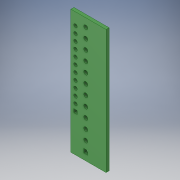
# Autodesk Inventor part: 3_5MM_TO_5_08MM_ADAPTOR_PCB
Saved by Autodesk Inventor 2018 (Build 220112000, 112)
## iProperties
Created: 2018-09-24
Part Number: 3_5MM_TO_5_08MM_ADAPTOR_PCB
Material: ABS Plastic
Document SubType Name: Modeling
Designer: Rich
Density: 1.06 g/cm^3
Appearance: Smooth - Dark Forest Green
Author: Rich
Autodesk Inventor part; units mm, degrees
(part 1 of 13)
ref_plane "YZ Plane" through (0, 0, 0) normal (1, 0, 0) x (0, 1, 0)
ref_plane "XZ Plane" through (0, 0, 0) normal (0, 1, 0) x (-1, 0, 0)
ref_plane "XY Plane" through (0, 0, 0) normal (0, 0, 1) x (1, 0, 0)
sketch "Sketch13" plane through (0, 0, 0) normal (0, 0, 1) x (1, 0, 0)
  line L0 (7.6746, 55.5524) -> (7.2, 55.5524)
  arc A0 (7.2, 55.5524) -> (7.2, 55.5016) centre (7.2, 55.527) ccw
  line L1 (7.7, 55.3688) -> (7.7, 55.6852)
  arc A1 (7.7, 55.6852) -> (7.6492, 55.6852) centre (7.6746, 55.6852) ccw
  line L2 (7.6492, 55.6852) -> (7.6492, 55.3688)
  arc A2 (7.6492, 55.3688) -> (7.7, 55.3688) centre (7.6746, 55.3688) ccw
  line L3 (7.3762, 59.9834) -> (7.218, 60.1416)
  arc A3 (7.218, 60.1416) -> (7.182, 60.1056) centre (7.2, 60.1236) ccw
  line L4 (7.182, 60.1056) -> (7.3402, 59.9474)
  arc A4 (7.3402, 59.9474) -> (7.3762, 59.9834) centre (7.3582, 59.9654) ccw
  line L5 (7.2, 60.0982) -> (7.6746, 60.0982)
  arc A5 (7.6746, 60.0982) -> (7.6746, 60.149) centre (7.6746, 60.1236) ccw
  line L6 (7.6746, 60.149) -> (7.2, 60.149)
  arc A6 (7.2, 60.149) -> (7.2, 60.0982) centre (7.2, 60.1236) ccw
  line L7 (7.7, 59.9654) -> (7.7, 60.2818)
  arc A7 (7.7, 60.2818) -> (7.6492, 60.2818) centre (7.6746, 60.2818) ccw
  line L8 (7.6492, 60.2818) -> (7.6492, 59.9654)
  arc A8 (7.6492, 59.9654) -> (7.7, 59.9654) centre (7.6746, 59.9654) ccw
  line L9 (7.6492, 60.7652) -> (7.6492, 60.4488)
  arc A9 (7.6492, 60.4488) -> (7.7, 60.4488) centre (7.6746, 60.4488) ccw
  line L10 (7.7, 60.4488) -> (7.7, 60.7652)
  arc A10 (7.7, 60.7652) -> (7.6492, 60.7652) centre (7.6746, 60.7661) ccw
  line L11 (7.6926, 60.4668) -> (7.3762, 60.7832)
  arc A11 (7.3762, 60.7832) -> (7.3402, 60.7472) centre (7.3582, 60.7652) ccw
  line L12 (7.3402, 60.7472) -> (7.6566, 60.4308)
  arc A12 (7.6566, 60.4308) -> (7.6926, 60.4668) centre (7.6746, 60.4488) ccw
  line L13 (7.3582, 60.7906) -> (7.2791, 60.7906)
  arc A13 (7.2791, 60.7906) -> (7.2791, 60.7398) centre (7.2791, 60.7652) ccw
  line L14 (7.2791, 60.7398) -> (7.3582, 60.7398)
  arc A14 (7.3582, 60.7398) -> (7.3582, 60.7906) centre (7.3582, 60.7652) ccw
  line L15 (7.2611, 60.7832) -> (7.182, 60.7041)
  arc A15 (7.182, 60.7041) -> (7.218, 60.6681) centre (7.2, 60.6861) ccw
  line L16 (7.218, 60.6681) -> (7.2971, 60.7472)
  arc A16 (7.2971, 60.7472) -> (7.2611, 60.7832) centre (7.2791, 60.7652) ccw
  line L17 (7.1746, 60.6861) -> (7.1746, 60.5279)
  arc A17 (7.1746, 60.5279) -> (7.2254, 60.5279) centre (7.2, 60.5279) ccw
  line L18 (7.2254, 60.5279) -> (7.2254, 60.6861)
  arc A18 (7.2254, 60.6861) -> (7.1746, 60.6861) centre (7.2, 60.6861) ccw
  line L19 (7.182, 60.5099) -> (7.2611, 60.4308)
  arc A19 (7.2611, 60.4308) -> (7.2971, 60.4668) centre (7.2791, 60.4488) ccw
  line L20 (7.2971, 60.4668) -> (7.218, 60.5459)
  arc A20 (7.218, 60.5459) -> (7.182, 60.5099) centre (7.2, 60.5279) ccw
  line L21 (7.3762, 4.1034) -> (7.218, 4.2616)
  arc A21 (7.218, 4.2616) -> (7.182, 4.2256) centre (7.2, 4.2436) ccw
  line L22 (7.182, 4.2256) -> (7.3402, 4.0674)
  arc A22 (7.3402, 4.0674) -> (7.3762, 4.1034) centre (7.3582, 4.0854) ccw
  line L23 (7.2, 4.2182) -> (7.6746, 4.2182)
  arc A23 (7.6746, 4.2182) -> (7.6746, 4.269) centre (7.6746, 4.2436) ccw
  line L24 (7.6746, 4.269) -> (7.2, 4.269)
  arc A24 (7.2, 4.269) -> (7.2, 4.2182) centre (7.2, 4.2436) ccw
  line L25 (7.7, 4.0854) -> (7.7, 4.4018)
  arc A25 (7.7, 4.4018) -> (7.6492, 4.4018) centre (7.6746, 4.4018) ccw
  line L26 (7.6492, 4.4018) -> (7.6492, 4.0854)
  arc A26 (7.6492, 4.0854) -> (7.7, 4.0854) centre (7.6746, 4.0854) ccw
  line L27 (7.6492, 9.4818) -> (7.6492, 9.1654)
  arc A27 (7.6492, 9.1654) -> (7.7, 9.1654) centre (7.6746, 9.1654) ccw
  line L28 (7.7, 9.1654) -> (7.7, 9.4818)
  arc A28 (7.7, 9.4818) -> (7.6492, 9.4818) centre (7.6746, 9.4827) ccw
  line L29 (7.6926, 9.1834) -> (7.3762, 9.4998)
  arc A29 (7.3762, 9.4998) -> (7.3402, 9.4638) centre (7.3582, 9.4818) ccw
  line L30 (7.3402, 9.4638) -> (7.6566, 9.1474)
  arc A30 (7.6566, 9.1474) -> (7.6926, 9.1834) centre (7.6746, 9.1654) ccw
  line L31 (7.3582, 9.5072) -> (7.2791, 9.5072)
  arc A31 (7.2791, 9.5072) -> (7.2791, 9.4564) centre (7.2791, 9.4818) ccw
  line L32 (7.2791, 9.4564) -> (7.3582, 9.4564)
  arc A32 (7.3582, 9.4564) -> (7.3582, 9.5072) centre (7.3582, 9.4818) ccw
  line L33 (7.2611, 9.4998) -> (7.182, 9.4207)
  arc A33 (7.182, 9.4207) -> (7.218, 9.3847) centre (7.2, 9.4027) ccw
  line L34 (7.218, 9.3847) -> (7.2971, 9.4638)
  arc A34 (7.2971, 9.4638) -> (7.2611, 9.4998) centre (7.2791, 9.4818) ccw
  line L35 (7.1746, 9.4027) -> (7.1746, 9.2445)
  arc A35 (7.1746, 9.2445) -> (7.2254, 9.2445) centre (7.2, 9.2445) ccw
  line L36 (7.2254, 9.2445) -> (7.2254, 9.4027)
  arc A36 (7.2254, 9.4027) -> (7.1746, 9.4027) centre (7.2, 9.4027) ccw
  line L37 (7.182, 9.2265) -> (7.2611, 9.1474)
  arc A37 (7.2611, 9.1474) -> (7.2971, 9.1834) centre (7.2791, 9.1654) ccw
  line L38 (7.2971, 9.1834) -> (7.218, 9.2625)
  arc A38 (7.218, 9.2625) -> (7.182, 9.2265) centre (7.2, 9.2445) ccw
  line L39 (7.2971, 14.2634) -> (7.218, 14.3425)
  arc A39 (7.218, 14.3425) -> (7.182, 14.3065) centre (7.2, 14.3245) ccw
  line L40 (7.182, 14.3065) -> (7.2611, 14.2274)
  arc A40 (7.2611, 14.2274) -> (7.2971, 14.2634) centre (7.2791, 14.2454) ccw
  line L41 (7.2254, 14.3245) -> (7.2254, 14.4827)
  arc A41 (7.2254, 14.4827) -> (7.1746, 14.4827) centre (7.2, 14.4827) ccw
  line L42 (7.1746, 14.4827) -> (7.1746, 14.3245)
  arc A42 (7.1746, 14.3245) -> (7.2254, 14.3245) centre (7.2, 14.3245) ccw
  line L43 (7.218, 14.4647) -> (7.2971, 14.5438)
  arc A43 (7.2971, 14.5438) -> (7.2611, 14.5798) centre (7.2791, 14.5618) ccw
  line L44 (7.2611, 14.5798) -> (7.182, 14.5007)
  arc A44 (7.182, 14.5007) -> (7.218, 14.4647) centre (7.2, 14.4827) ccw
  line L45 (7.2791, 14.5364) -> (7.3582, 14.5364)
  arc A45 (7.3582, 14.5364) -> (7.3582, 14.5872) centre (7.3582, 14.5618) ccw
  line L46 (7.3582, 14.5872) -> (7.2791, 14.5872)
  arc A46 (7.2791, 14.5872) -> (7.2791, 14.5364) centre (7.2791, 14.5618) ccw
  line L47 (7.3402, 14.5438) -> (7.4193, 14.4647)
  arc A47 (7.4193, 14.4647) -> (7.4553, 14.5007) centre (7.4373, 14.4827) ccw
  line L48 (7.4553, 14.5007) -> (7.3762, 14.5798)
  arc A48 (7.3762, 14.5798) -> (7.3402, 14.5438) centre (7.3582, 14.5618) ccw
  line L49 (7.4119, 14.4827) -> (7.4119, 14.4036)
  arc A49 (7.4119, 14.4036) -> (7.4627, 14.4036) centre (7.4373, 14.4036) ccw
  line L50 (7.4627, 14.4036) -> (7.4627, 14.4827)
  arc A50 (7.4627, 14.4827) -> (7.4119, 14.4827) centre (7.4373, 14.4827) ccw
  line L51 (7.4553, 14.4647) -> (7.5344, 14.5438)
  arc A51 (7.5344, 14.5438) -> (7.4984, 14.5798) centre (7.5164, 14.5618) ccw
  line L52 (7.4984, 14.5798) -> (7.4193, 14.5007)
  arc A52 (7.4193, 14.5007) -> (7.4553, 14.4647) centre (7.4373, 14.4827) ccw
  line L53 (7.5164, 14.5364) -> (7.5955, 14.5364)
  arc A53 (7.5955, 14.5364) -> (7.5955, 14.5872) centre (7.5955, 14.5618) ccw
  line L54 (7.5955, 14.5872) -> (7.5164, 14.5872)
  arc A54 (7.5164, 14.5872) -> (7.5164, 14.5364) centre (7.5164, 14.5618) ccw
  line L55 (7.5775, 14.5438) -> (7.6566, 14.4647)
  arc A55 (7.6566, 14.4647) -> (7.6926, 14.5007) centre (7.6746, 14.4827) ccw
  line L56 (7.6926, 14.5007) -> (7.6135, 14.5798)
  arc A56 (7.6135, 14.5798) -> (7.5775, 14.5438) centre (7.5955, 14.5618) ccw
  line L57 (7.6492, 14.4827) -> (7.6492, 14.3245)
  arc A57 (7.6492, 14.3245) -> (7.7, 14.3245) centre (7.6746, 14.3245) ccw
  line L58 (7.7, 14.3245) -> (7.7, 14.4827)
  arc A58 (7.7, 14.4827) -> (7.6492, 14.4827) centre (7.6746, 14.4827) ccw
  line L59 (7.6566, 14.3425) -> (7.5775, 14.2634)
  arc A59 (7.5775, 14.2634) -> (7.6135, 14.2274) centre (7.5955, 14.2454) ccw
  line L60 (7.6135, 14.2274) -> (7.6926, 14.3065)
  arc A60 (7.6926, 14.3065) -> (7.6566, 14.3425) centre (7.6746, 14.3245) ccw
  line L61 (7.6746, 19.5881) -> (7.2, 19.5881)
  arc A61 (7.2, 19.5881) -> (7.2, 19.5373) centre (7.2, 19.5627) ccw
  line L62 (7.2, 19.5373) -> (7.6746, 19.5373)
  arc A62 (7.6746, 19.5373) -> (7.6746, 19.5881) centre (7.6746, 19.5627) ccw
  line L63 (7.182, 19.5447) -> (7.4193, 19.3074)
  arc A63 (7.4193, 19.3074) -> (7.4553, 19.3434) centre (7.4373, 19.3254) ccw
  line L64 (7.4553, 19.3434) -> (7.218, 19.5807)
  arc A64 (7.218, 19.5807) -> (7.182, 19.5447) centre (7.2, 19.5627) ccw
  line L65 (7.4627, 19.3254) -> (7.4627, 19.6418)
  arc A65 (7.4627, 19.6418) -> (7.4119, 19.6418) centre (7.4373, 19.6418) ccw
  line L66 (7.4119, 19.6418) -> (7.4119, 19.3254)
  arc A66 (7.4119, 19.3254) -> (7.4627, 19.3254) centre (7.4373, 19.3254) ccw
  line L67 (7.1746, 24.7218) -> (7.1746, 24.4054)
  arc A67 (7.1746, 24.4054) -> (7.2254, 24.4054) centre (7.2, 24.4054) ccw
  line L68 (7.2254, 24.4054) -> (7.2254, 24.7218)
  arc A68 (7.2254, 24.7218) -> (7.1746, 24.7218) centre (7.2, 24.7218) ccw
  line L69 (7.2, 24.38) -> (7.4373, 24.38)
  arc A69 (7.4373, 24.38) -> (7.4373, 24.4308) centre (7.4373, 24.4054) ccw
  line L70 (7.4373, 24.4308) -> (7.2, 24.4308)
  arc A70 (7.2, 24.4308) -> (7.2, 24.38) centre (7.2, 24.4054) ccw
  line L71 (7.46, 24.4168) -> (7.3809, 24.575)
  arc A71 (7.3809, 24.575) -> (7.3355, 24.5522) centre (7.3582, 24.5636) ccw
  line L72 (7.3355, 24.5522) -> (7.4146, 24.394)
  arc A72 (7.4146, 24.394) -> (7.46, 24.4168) centre (7.4373, 24.4054) ccw
  line L73 (7.3836, 24.5636) -> (7.3836, 24.6427)
  arc A73 (7.3836, 24.6427) -> (7.3328, 24.6427) centre (7.3582, 24.6427) ccw
  line L74 (7.3328, 24.6427) -> (7.3328, 24.5636)
  arc A74 (7.3328, 24.5636) -> (7.3836, 24.5636) centre (7.3582, 24.5636) ccw
  line L75 (7.3762, 24.6247) -> (7.4553, 24.7038)
  arc A75 (7.4553, 24.7038) -> (7.4193, 24.7398) centre (7.4373, 24.7218) ccw
  line L76 (7.4193, 24.7398) -> (7.3402, 24.6607)
  arc A76 (7.3402, 24.6607) -> (7.3762, 24.6247) centre (7.3582, 24.6427) ccw
  line L77 (7.4373, 24.6964) -> (7.5955, 24.6964)
  arc A77 (7.5955, 24.6964) -> (7.5955, 24.7472) centre (7.5955, 24.7218) ccw
  line L78 (7.5955, 24.7472) -> (7.4373, 24.7472)
  arc A78 (7.4373, 24.7472) -> (7.4373, 24.6964) centre (7.4373, 24.7218) ccw
  line L79 (7.5775, 24.7038) -> (7.6566, 24.6247)
  arc A79 (7.6566, 24.6247) -> (7.6926, 24.6607) centre (7.6746, 24.6427) ccw
  line L80 (7.6926, 24.6607) -> (7.6135, 24.7398)
  arc A80 (7.6135, 24.7398) -> (7.5775, 24.7038) centre (7.5955, 24.7218) ccw
  line L81 (7.6492, 24.6427) -> (7.6492, 24.4845)
  arc A81 (7.6492, 24.4845) -> (7.7, 24.4845) centre (7.6746, 24.4845) ccw
  line L82 (7.7, 24.4845) -> (7.7, 24.6427)
  arc A82 (7.7, 24.6427) -> (7.6492, 24.6427) centre (7.6746, 24.6427) ccw
  line L83 (7.6566, 24.5025) -> (7.5775, 24.4234)
  arc A83 (7.5775, 24.4234) -> (7.6135, 24.3874) centre (7.5955, 24.4054) ccw
  line L84 (7.6135, 24.3874) -> (7.6926, 24.4665)
  arc A84 (7.6926, 24.4665) -> (7.6566, 24.5025) centre (7.6746, 24.4845) ccw
  line L85 (7.1773, 29.7904) -> (7.2564, 29.6322)
  arc A85 (7.2564, 29.6322) -> (7.3018, 29.655) centre (7.2791, 29.6436) ccw
  line L86 (7.3018, 29.655) -> (7.2227, 29.8132)
  arc A86 (7.2227, 29.8132) -> (7.1773, 29.7904) centre (7.2, 29.8018) ccw
  line L87 (7.2611, 29.6256) -> (7.4193, 29.4674)
  arc A87 (7.4193, 29.4674) -> (7.4553, 29.5034) centre (7.4373, 29.4854) ccw
  line L88 (7.4553, 29.5034) -> (7.2971, 29.6616)
  arc A88 (7.2971, 29.6616) -> (7.2611, 29.6256) centre (7.2791, 29.6436) ccw
  line L89 (7.4373, 29.46) -> (7.5955, 29.46)
  arc A89 (7.5955, 29.46) -> (7.5955, 29.5108) centre (7.5955, 29.4854) ccw
  line L90 (7.5955, 29.5108) -> (7.4373, 29.5108)
  arc A90 (7.4373, 29.5108) -> (7.4373, 29.46) centre (7.4373, 29.4854) ccw
  line L91 (7.6135, 29.4674) -> (7.6926, 29.5465)
  arc A91 (7.6926, 29.5465) -> (7.6566, 29.5825) centre (7.6746, 29.5645) ccw
  line L92 (7.6566, 29.5825) -> (7.5775, 29.5034)
  arc A92 (7.5775, 29.5034) -> (7.6135, 29.4674) centre (7.5955, 29.4854) ccw
  line L93 (7.7, 29.5645) -> (7.7, 29.7227)
  arc A93 (7.7, 29.7227) -> (7.6492, 29.7227) centre (7.6746, 29.7227) ccw
  line L94 (7.6492, 29.7227) -> (7.6492, 29.5645)
  arc A94 (7.6492, 29.5645) -> (7.7, 29.5645) centre (7.6746, 29.5645) ccw
  line L95 (7.6926, 29.7407) -> (7.6135, 29.8198)
  arc A95 (7.6135, 29.8198) -> (7.5775, 29.7838) centre (7.5955, 29.8018) ccw
  line L96 (7.5775, 29.7838) -> (7.6566, 29.7047)
  arc A96 (7.6566, 29.7047) -> (7.6926, 29.7407) centre (7.6746, 29.7227) ccw
  line L97 (7.5955, 29.8272) -> (7.5164, 29.8272)
  arc A97 (7.5164, 29.8272) -> (7.5164, 29.7764) centre (7.5164, 29.8018) ccw
  line L98 (7.5164, 29.7764) -> (7.5955, 29.7764)
  arc A98 (7.5955, 29.7764) -> (7.5955, 29.8272) centre (7.5955, 29.8018) ccw
  line L99 (7.4984, 29.8198) -> (7.4193, 29.7407)
  arc A99 (7.4193, 29.7407) -> (7.4553, 29.7047) centre (7.4373, 29.7227) ccw
  line L100 (7.4553, 29.7047) -> (7.5344, 29.7838)
  arc A100 (7.5344, 29.7838) -> (7.4984, 29.8198) centre (7.5164, 29.8018) ccw
  line L101 (7.4119, 29.7227) -> (7.4119, 29.4854)
  arc A101 (7.4119, 29.4854) -> (7.4627, 29.4854) centre (7.4373, 29.4854) ccw
  line L102 (7.4627, 29.4854) -> (7.4627, 29.7227)
  arc A102 (7.4627, 29.7227) -> (7.4119, 29.7227) centre (7.4373, 29.7227) ccw
  line L103 (7.2254, 34.5654) -> (7.2254, 34.8818)
  arc A103 (7.2254, 34.8818) -> (7.1746, 34.8818) centre (7.2, 34.8818) ccw
  line L104 (7.1746, 34.8818) -> (7.1746, 34.5654)
  arc A104 (7.1746, 34.5654) -> (7.2254, 34.5654) centre (7.2, 34.5654) ccw
  line L105 (7.2, 34.8564) -> (7.2791, 34.8564)
  arc A105 (7.2791, 34.8564) -> (7.2791, 34.9072) centre (7.2791, 34.8818) ccw
  line L106 (7.2791, 34.9072) -> (7.2, 34.9072)
  arc A106 (7.2, 34.9072) -> (7.2, 34.8564) centre (7.2, 34.8818) ccw
  line L107 (7.2611, 34.8638) -> (7.5775, 34.5474)
  arc A107 (7.5775, 34.5474) -> (7.6135, 34.5834) centre (7.5955, 34.5654) ccw
  line L108 (7.6135, 34.5834) -> (7.2971, 34.8998)
  arc A108 (7.2971, 34.8998) -> (7.2611, 34.8638) centre (7.2791, 34.8818) ccw
  line L109 (7.5955, 34.54) -> (7.6746, 34.54)
  arc A109 (7.6746, 34.54) -> (7.6746, 34.5908) centre (7.6746, 34.5654) ccw
  line L110 (7.6746, 34.5908) -> (7.5955, 34.5908)
  arc A110 (7.5955, 34.5908) -> (7.5955, 34.54) centre (7.5955, 34.5654) ccw
  line L111 (7.2971, 39.6634) -> (7.218, 39.7425)
  arc A111 (7.218, 39.7425) -> (7.182, 39.7065) centre (7.2, 39.7245) ccw
  line L112 (7.182, 39.7065) -> (7.2611, 39.6274)
  arc A112 (7.2611, 39.6274) -> (7.2971, 39.6634) centre (7.2791, 39.6454) ccw
  line L113 (7.2254, 39.7245) -> (7.2254, 39.8827)
  arc A113 (7.2254, 39.8827) -> (7.1746, 39.8827) centre (7.2, 39.8827) ccw
  line L114 (7.1746, 39.8827) -> (7.1746, 39.7245)
  arc A114 (7.1746, 39.7245) -> (7.2254, 39.7245) centre (7.2, 39.7245) ccw
  line L115 (7.218, 39.8647) -> (7.2971, 39.9438)
  arc A115 (7.2971, 39.9438) -> (7.2611, 39.9798) centre (7.2791, 39.9618) ccw
  line L116 (7.2611, 39.9798) -> (7.182, 39.9007)
  arc A116 (7.182, 39.9007) -> (7.218, 39.8647) centre (7.2, 39.8827) ccw
  line L117 (7.2791, 39.9364) -> (7.3582, 39.9364)
  arc A117 (7.3582, 39.9364) -> (7.3582, 39.9872) centre (7.3582, 39.9618) ccw
  line L118 (7.3582, 39.9872) -> (7.2791, 39.9872)
  arc A118 (7.2791, 39.9872) -> (7.2791, 39.9364) centre (7.2791, 39.9618) ccw
  line L119 (7.3402, 39.9438) -> (7.4193, 39.8647)
  arc A119 (7.4193, 39.8647) -> (7.4553, 39.9007) centre (7.4373, 39.8827) ccw
  line L120 (7.4553, 39.9007) -> (7.3762, 39.9798)
  arc A120 (7.3762, 39.9798) -> (7.3402, 39.9438) centre (7.3582, 39.9618) ccw
  line L121 (7.4553, 39.8647) -> (7.5344, 39.9438)
  arc A121 (7.5344, 39.9438) -> (7.4984, 39.9798) centre (7.5164, 39.9618) ccw
  line L122 (7.4984, 39.9798) -> (7.4193, 39.9007)
  arc A122 (7.4193, 39.9007) -> (7.4553, 39.8647) centre (7.4373, 39.8827) ccw
  line L123 (7.5164, 39.9364) -> (7.5955, 39.9364)
  arc A123 (7.5955, 39.9364) -> (7.5955, 39.9872) centre (7.5955, 39.9618) ccw
  line L124 (7.5955, 39.9872) -> (7.5164, 39.9872)
  arc A124 (7.5164, 39.9872) -> (7.5164, 39.9364) centre (7.5164, 39.9618) ccw
  line L125 (7.5775, 39.9438) -> (7.6566, 39.8647)
  arc A125 (7.6566, 39.8647) -> (7.6926, 39.9007) centre (7.6746, 39.8827) ccw
  line L126 (7.6926, 39.9007) -> (7.6135, 39.9798)
  arc A126 (7.6135, 39.9798) -> (7.5775, 39.9438) centre (7.5955, 39.9618) ccw
  line L127 (7.6492, 39.8827) -> (7.6492, 39.7245)
  arc A127 (7.6492, 39.7245) -> (7.7, 39.7245) centre (7.6746, 39.7245) ccw
  line L128 (7.7, 39.7245) -> (7.7, 39.8827)
  arc A128 (7.7, 39.8827) -> (7.6492, 39.8827) centre (7.6746, 39.8827) ccw
  line L129 (7.6566, 39.7425) -> (7.5775, 39.6634)
  arc A129 (7.5775, 39.6634) -> (7.6135, 39.6274) centre (7.5955, 39.6454) ccw
  line L130 (7.6135, 39.6274) -> (7.6926, 39.7065)
  arc A130 (7.6926, 39.7065) -> (7.6566, 39.7425) centre (7.6746, 39.7245) ccw
  line L131 (7.5955, 39.6708) -> (7.5164, 39.6708)
  arc A131 (7.5164, 39.6708) -> (7.5164, 39.62) centre (7.5164, 39.6454) ccw
  line L132 (7.5164, 39.62) -> (7.5955, 39.62)
  arc A132 (7.5955, 39.62) -> (7.5955, 39.6708) centre (7.5955, 39.6454) ccw
  line L133 (7.5344, 39.6634) -> (7.4553, 39.7425)
  arc A133 (7.4553, 39.7425) -> (7.4193, 39.7065) centre (7.4373, 39.7245) ccw
  line L134 (7.4193, 39.7065) -> (7.4984, 39.6274)
  arc A134 (7.4984, 39.6274) -> (7.5344, 39.6634) centre (7.5164, 39.6454) ccw
  line L135 (7.4193, 39.7425) -> (7.3402, 39.6634)
  arc A135 (7.3402, 39.6634) -> (7.3762, 39.6274) centre (7.3582, 39.6454) ccw
  line L136 (7.3762, 39.6274) -> (7.4553, 39.7065)
  arc A136 (7.4553, 39.7065) -> (7.4193, 39.7425) centre (7.4373, 39.7245) ccw
  line L137 (7.3582, 39.6708) -> (7.2791, 39.6708)
  arc A137 (7.2791, 39.6708) -> (7.2791, 39.62) centre (7.2791, 39.6454) ccw
  line L138 (7.2791, 39.62) -> (7.3582, 39.62)
  arc A138 (7.3582, 39.62) -> (7.3582, 39.6708) centre (7.3582, 39.6454) ccw
  line L139 (7.4627, 39.7245) -> (7.4627, 39.8827)
  arc A139 (7.4627, 39.8827) -> (7.4119, 39.8827) centre (7.4373, 39.8827) ccw
  line L140 (7.4119, 39.8827) -> (7.4119, 39.7245)
  arc A140 (7.4119, 39.7245) -> (7.4627, 39.7245) centre (7.4373, 39.7245) ccw
  line L141 (7.6135, 44.7074) -> (7.6926, 44.7865)
  arc A141 (7.6926, 44.7865) -> (7.6566, 44.8225) centre (7.6746, 44.8045) ccw
  line L142 (7.6566, 44.8225) -> (7.5775, 44.7434)
  arc A142 (7.5775, 44.7434) -> (7.6135, 44.7074) centre (7.5955, 44.7254) ccw
  line L143 (7.7, 44.8045) -> (7.7, 44.9627)
  arc A143 (7.7, 44.9627) -> (7.6492, 44.9627) centre (7.6746, 44.9627) ccw
  line L144 (7.6492, 44.9627) -> (7.6492, 44.8045)
  arc A144 (7.6492, 44.8045) -> (7.7, 44.8045) centre (7.6746, 44.8045) ccw
  line L145 (7.6926, 44.9807) -> (7.6135, 45.0598)
  arc A145 (7.6135, 45.0598) -> (7.5775, 45.0238) centre (7.5955, 45.0418) ccw
  line L146 (7.5775, 45.0238) -> (7.6566, 44.9447)
  arc A146 (7.6566, 44.9447) -> (7.6926, 44.9807) centre (7.6746, 44.9627) ccw
  line L147 (7.5955, 45.0672) -> (7.2791, 45.0672)
  arc A147 (7.2791, 45.0672) -> (7.2791, 45.0164) centre (7.2791, 45.0418) ccw
  line L148 (7.2791, 45.0164) -> (7.5955, 45.0164)
  arc A148 (7.5955, 45.0164) -> (7.5955, 45.0672) centre (7.5955, 45.0418) ccw
  line L149 (7.2611, 45.0598) -> (7.182, 44.9807)
  arc A149 (7.182, 44.9807) -> (7.218, 44.9447) centre (7.2, 44.9627) ccw
  line L150 (7.218, 44.9447) -> (7.2971, 45.0238)
  arc A150 (7.2971, 45.0238) -> (7.2611, 45.0598) centre (7.2791, 45.0418) ccw
  line L151 (7.1746, 44.9627) -> (7.1746, 44.8045)
  arc A151 (7.1746, 44.8045) -> (7.2254, 44.8045) centre (7.2, 44.8045) ccw
  line L152 (7.2254, 44.8045) -> (7.2254, 44.9627)
  arc A152 (7.2254, 44.9627) -> (7.1746, 44.9627) centre (7.2, 44.9627) ccw
  line L153 (7.182, 44.7865) -> (7.2611, 44.7074)
  arc A153 (7.2611, 44.7074) -> (7.2971, 44.7434) centre (7.2791, 44.7254) ccw
  line L154 (7.2971, 44.7434) -> (7.218, 44.8225)
  arc A154 (7.218, 44.8225) -> (7.182, 44.7865) centre (7.2, 44.8045) ccw
  line L155 (7.2791, 44.7) -> (7.3582, 44.7)
  arc A155 (7.3582, 44.7) -> (7.3582, 44.7508) centre (7.3582, 44.7254) ccw
  line L156 (7.3582, 44.7508) -> (7.2791, 44.7508)
  arc A156 (7.2791, 44.7508) -> (7.2791, 44.7) centre (7.2791, 44.7254) ccw
  line L157 (7.3762, 44.7074) -> (7.4553, 44.7865)
  arc A157 (7.4553, 44.7865) -> (7.4193, 44.8225) centre (7.4373, 44.8045) ccw
  line L158 (7.4193, 44.8225) -> (7.3402, 44.7434)
  arc A158 (7.3402, 44.7434) -> (7.3762, 44.7074) centre (7.3582, 44.7254) ccw
  line L159 (7.4627, 44.8045) -> (7.4627, 45.0418)
  arc A159 (7.4627, 45.0418) -> (7.4119, 45.0418) centre (7.4373, 45.0418) ccw
  line L160 (7.4119, 45.0418) -> (7.4119, 44.8045)
  arc A160 (7.4119, 44.8045) -> (7.4627, 44.8045) centre (7.4373, 44.8045) ccw
  line L161 (7.3762, 49.8234) -> (7.218, 49.9816)
  arc A161 (7.218, 49.9816) -> (7.182, 49.9456) centre (7.2, 49.9636) ccw
  line L162 (7.182, 49.9456) -> (7.3402, 49.7874)
  arc A162 (7.3402, 49.7874) -> (7.3762, 49.8234) centre (7.3582, 49.8054) ccw
  line L163 (7.2, 49.9382) -> (7.6746, 49.9382)
  arc A163 (7.6746, 49.9382) -> (7.6746, 49.989) centre (7.6746, 49.9636) ccw
  line L164 (7.6746, 49.989) -> (7.2, 49.989)
  arc A164 (7.2, 49.989) -> (7.2, 49.9382) centre (7.2, 49.9636) ccw
  line L165 (7.7, 49.8054) -> (7.7, 50.1218)
  arc A165 (7.7, 50.1218) -> (7.6492, 50.1218) centre (7.6746, 50.1218) ccw
  line L166 (7.6492, 50.1218) -> (7.6492, 49.8054)
  arc A166 (7.6492, 49.8054) -> (7.7, 49.8054) centre (7.6746, 49.8054) ccw
  line L167 (7.5955, 50.3142) -> (7.2791, 50.3142)
  arc A167 (7.2791, 50.3142) -> (7.2791, 50.2634) centre (7.2791, 50.2888) ccw
  line L168 (7.2791, 50.2634) -> (7.5955, 50.2634)
  arc A168 (7.5955, 50.2634) -> (7.5955, 50.3142) centre (7.5955, 50.2888) ccw
  line L169 (7.2971, 50.3068) -> (7.218, 50.3859)
  arc A169 (7.218, 50.3859) -> (7.182, 50.3499) centre (7.2, 50.3679) ccw
  line L170 (7.182, 50.3499) -> (7.2611, 50.2708)
  arc A170 (7.2611, 50.2708) -> (7.2971, 50.3068) centre (7.2791, 50.2888) ccw
  line L171 (7.2254, 50.3679) -> (7.2254, 50.5261)
  arc A171 (7.2254, 50.5261) -> (7.1746, 50.5261) centre (7.2, 50.5261) ccw
  line L172 (7.1746, 50.5261) -> (7.1746, 50.3679)
  arc A172 (7.1746, 50.3679) -> (7.2254, 50.3679) centre (7.2, 50.3679) ccw
  line L173 (7.218, 50.5081) -> (7.2971, 50.5872)
  arc A173 (7.2971, 50.5872) -> (7.2611, 50.6232) centre (7.2791, 50.6052) ccw
  line L174 (7.2611, 50.6232) -> (7.182, 50.5441)
  arc A174 (7.182, 50.5441) -> (7.218, 50.5081) centre (7.2, 50.5261) ccw
  line L175 (7.2791, 50.5798) -> (7.5955, 50.5798)
  arc A175 (7.5955, 50.5798) -> (7.5955, 50.6306) centre (7.5955, 50.6052) ccw
  line L176 (7.5955, 50.6306) -> (7.2791, 50.6306)
  arc A176 (7.2791, 50.6306) -> (7.2791, 50.5798) centre (7.2791, 50.6052) ccw
  line L177 (7.5775, 50.5872) -> (7.6566, 50.5081)
  arc A177 (7.6566, 50.5081) -> (7.6926, 50.5441) centre (7.6746, 50.5261) ccw
  line L178 (7.6926, 50.5441) -> (7.6135, 50.6232)
  arc A178 (7.6135, 50.6232) -> (7.5775, 50.5872) centre (7.5955, 50.6052) ccw
  line L179 (7.6492, 50.5261) -> (7.6492, 50.3679)
  arc A179 (7.6492, 50.3679) -> (7.7, 50.3679) centre (7.6746, 50.3679) ccw
  line L180 (7.7, 50.3679) -> (7.7, 50.5261)
  arc A180 (7.7, 50.5261) -> (7.6492, 50.5261) centre (7.6746, 50.5261) ccw
  line L181 (7.6566, 50.3859) -> (7.5775, 50.3068)
  arc A181 (7.5775, 50.3068) -> (7.6135, 50.2708) centre (7.5955, 50.2888) ccw
  line L182 (7.6135, 50.2708) -> (7.6926, 50.3499)
  arc A182 (7.6926, 50.3499) -> (7.6566, 50.3859) centre (7.6746, 50.3679) ccw
  line L183 (7.6135, 50.3068) -> (7.2971, 50.6232)
  arc A183 (7.2971, 50.6232) -> (7.2611, 50.5872) centre (7.2791, 50.6052) ccw
  line L184 (7.2611, 50.5872) -> (7.5775, 50.2708)
  arc A184 (7.5775, 50.2708) -> (7.6135, 50.3068) centre (7.5955, 50.2888) ccw
  line L185 (7.3762, 54.9034) -> (7.218, 55.0616)
  arc A185 (7.218, 55.0616) -> (7.182, 55.0256) centre (7.2, 55.0436) ccw
  line L186 (7.182, 55.0256) -> (7.3402, 54.8674)
  arc A186 (7.3402, 54.8674) -> (7.3762, 54.9034) centre (7.3582, 54.8854) ccw
  line L187 (7.2, 55.0182) -> (7.6746, 55.0182)
  arc A187 (7.6746, 55.0182) -> (7.6746, 55.069) centre (7.6746, 55.0436) ccw
  line L188 (7.6746, 55.069) -> (7.2, 55.069)
  arc A188 (7.2, 55.069) -> (7.2, 55.0182) centre (7.2, 55.0436) ccw
  line L189 (7.7, 54.8854) -> (7.7, 55.2018)
  arc A189 (7.7, 55.2018) -> (7.6492, 55.2018) centre (7.6746, 55.2018) ccw
  line L190 (7.6492, 55.2018) -> (7.6492, 54.8854)
  arc A190 (7.6492, 54.8854) -> (7.7, 54.8854) centre (7.6746, 54.8854) ccw
  line L191 (7.3762, 55.3868) -> (7.218, 55.545)
  arc A191 (7.218, 55.545) -> (7.182, 55.509) centre (7.2, 55.527) ccw
  line L192 (7.182, 55.509) -> (7.3402, 55.3508)
  arc A192 (7.3402, 55.3508) -> (7.3762, 55.3868) centre (7.3582, 55.3688) ccw
  line L193 (7.2, 55.5016) -> (7.6746, 55.5016)
  arc A193 (7.6746, 55.5016) -> (7.6746, 55.5524) centre (7.6746, 55.527) ccw
  line L194 (17.121, 38.367) -> (8.095, 38.367)
  arc A194 (8.095, 38.367) -> (8.095, 38.241) centre (8.095, 38.304) ccw
  line L195 (1.0789, 38.367) -> (7.0006, 38.367)
  arc A195 (7.0006, 38.367) -> (7.0006, 38.493) centre (7.0006, 38.43) ccw
  line L196 (7.0006, 38.493) -> (1.0789, 38.493)
  arc A196 (1.0789, 38.493) -> (1.0789, 38.367) centre (1.0789, 38.43) ccw
  line L197 (7.637, 38.367) -> (7.7628, 38.367)
  arc A197 (7.7628, 38.367) -> (7.7628, 38.493) centre (7.7628, 38.43) ccw
  line L198 (7.7628, 38.493) -> (7.637, 38.493)
  arc A198 (7.637, 38.493) -> (7.637, 38.367) centre (7.637, 38.43) ccw
  line L199 (8.3992, 38.367) -> (17.121, 38.367)
  arc A199 (17.121, 38.367) -> (17.121, 38.493) centre (17.121, 38.43) ccw
  line L200 (17.121, 38.493) -> (8.3992, 38.493)
  arc A200 (8.3992, 38.493) -> (8.3992, 38.367) centre (8.3992, 38.43) ccw
  line L201 (1.0789, 38.493) -> (6.8307, 38.493)
  arc A201 (6.8307, 38.493) -> (6.8307, 38.619) centre (6.8307, 38.556) ccw
  line L202 (6.8307, 38.619) -> (1.0789, 38.619)
  arc A202 (1.0789, 38.619) -> (1.0789, 38.493) centre (1.0789, 38.556) ccw
  line L203 (7.637, 38.493) -> (7.7628, 38.493)
  arc A203 (7.7628, 38.493) -> (7.7628, 38.619) centre (7.7628, 38.556) ccw
  line L204 (7.7628, 38.619) -> (7.637, 38.619)
  arc A204 (7.637, 38.619) -> (7.637, 38.493) centre (7.637, 38.556) ccw
  line L205 (8.5692, 38.493) -> (17.121, 38.493)
  arc A205 (17.121, 38.493) -> (17.121, 38.619) centre (17.121, 38.556) ccw
  line L206 (17.121, 38.619) -> (8.5692, 38.619)
  arc A206 (8.5692, 38.619) -> (8.5692, 38.493) centre (8.5692, 38.556) ccw
  line L207 (1.0789, 38.619) -> (6.7047, 38.619)
  arc A207 (6.7047, 38.619) -> (6.7047, 38.745) centre (6.7047, 38.682) ccw
  line L208 (6.7047, 38.745) -> (1.0789, 38.745)
  arc A208 (1.0789, 38.745) -> (1.0789, 38.619) centre (1.0789, 38.682) ccw
  line L209 (7.637, 38.619) -> (7.7628, 38.619)
  arc A209 (7.7628, 38.619) -> (7.7628, 38.745) centre (7.7628, 38.682) ccw
  line L210 (7.7628, 38.745) -> (7.637, 38.745)
  arc A210 (7.637, 38.745) -> (7.637, 38.619) centre (7.637, 38.682) ccw
  line L211 (8.6952, 38.619) -> (17.121, 38.619)
  arc A211 (17.121, 38.619) -> (17.121, 38.745) centre (17.121, 38.682) ccw
  line L212 (17.121, 38.745) -> (8.6952, 38.745)
  arc A212 (8.6952, 38.745) -> (8.6952, 38.619) centre (8.6952, 38.682) ccw
  line L213 (1.0789, 38.745) -> (6.5787, 38.745)
  arc A213 (6.5787, 38.745) -> (6.5787, 38.871) centre (6.5787, 38.808) ccw
  line L214 (6.5787, 38.871) -> (1.0789, 38.871)
  arc A214 (1.0789, 38.871) -> (1.0789, 38.745) centre (1.0789, 38.808) ccw
  line L215 (7.637, 38.745) -> (7.7628, 38.745)
  arc A215 (7.7628, 38.745) -> (7.7628, 38.871) centre (7.7628, 38.808) ccw
  line L216 (7.7628, 38.871) -> (7.637, 38.871)
  arc A216 (7.637, 38.871) -> (7.637, 38.745) centre (7.637, 38.808) ccw
  line L217 (8.8212, 38.745) -> (17.121, 38.745)
  arc A217 (17.121, 38.745) -> (17.121, 38.871) centre (17.121, 38.808) ccw
  line L218 (17.121, 38.871) -> (8.8212, 38.871)
  arc A218 (8.8212, 38.871) -> (8.8212, 38.745) centre (8.8212, 38.808) ccw
  line L219 (1.0789, 38.871) -> (6.5044, 38.871)
  arc A219 (6.5044, 38.871) -> (6.5044, 38.997) centre (6.5044, 38.934) ccw
  line L220 (6.5044, 38.997) -> (1.0789, 38.997)
  arc A220 (1.0789, 38.997) -> (1.0789, 38.871) centre (1.0789, 38.934) ccw
  line L221 (7.637, 38.871) -> (7.7628, 38.871)
  arc A221 (7.7628, 38.871) -> (7.7628, 38.997) centre (7.7628, 38.934) ccw
  line L222 (7.7628, 38.997) -> (7.637, 38.997)
  arc A222 (7.637, 38.997) -> (7.637, 38.871) centre (7.637, 38.934) ccw
  line L223 (8.8954, 38.871) -> (17.121, 38.871)
  arc A223 (17.121, 38.871) -> (17.121, 38.997) centre (17.121, 38.934) ccw
  line L224 (17.121, 38.997) -> (8.8954, 38.997)
  arc A224 (8.8954, 38.997) -> (8.8954, 38.871) centre (8.8954, 38.934) ccw
  line L225 (1.0789, 38.997) -> (6.4522, 38.997)
  arc A225 (6.4522, 38.997) -> (6.4522, 39.123) centre (6.4522, 39.06) ccw
  line L226 (6.4522, 39.123) -> (1.0789, 39.123)
  arc A226 (1.0789, 39.123) -> (1.0789, 38.997) centre (1.0789, 39.06) ccw
  line L227 (7.637, 38.997) -> (7.7628, 38.997)
  arc A227 (7.7628, 38.997) -> (7.7628, 39.123) centre (7.7628, 39.06) ccw
  line L228 (7.7628, 39.123) -> (7.637, 39.123)
  arc A228 (7.637, 39.123) -> (7.637, 38.997) centre (7.637, 39.06) ccw
  line L229 (8.9476, 38.997) -> (17.121, 38.997)
  arc A229 (17.121, 38.997) -> (17.121, 39.123) centre (17.121, 39.06) ccw
  line L230 (17.121, 39.123) -> (8.9476, 39.123)
  arc A230 (8.9476, 39.123) -> (8.9476, 38.997) centre (8.9476, 39.06) ccw
  line L231 (1.0789, 39.123) -> (6.4001, 39.123)
  arc A231 (6.4001, 39.123) -> (6.4001, 39.249) centre (6.4001, 39.186) ccw
  line L232 (6.4001, 39.249) -> (1.0789, 39.249)
  arc A232 (1.0789, 39.249) -> (1.0789, 39.123) centre (1.0789, 39.186) ccw
  line L233 (7.637, 39.123) -> (7.7628, 39.123)
  arc A233 (7.7628, 39.123) -> (7.7628, 39.249) centre (7.7628, 39.186) ccw
  line L234 (7.7628, 39.249) -> (7.637, 39.249)
  arc A234 (7.637, 39.249) -> (7.637, 39.123) centre (7.637, 39.186) ccw
  line L235 (8.9997, 39.123) -> (17.121, 39.123)
  arc A235 (17.121, 39.123) -> (17.121, 39.249) centre (17.121, 39.186) ccw
  line L236 (17.121, 39.249) -> (8.9997, 39.249)
  arc A236 (8.9997, 39.249) -> (8.9997, 39.123) centre (8.9997, 39.186) ccw
  line L237 (1.0789, 39.249) -> (6.3479, 39.249)
  arc A237 (6.3479, 39.249) -> (6.3479, 39.375) centre (6.3479, 39.312) ccw
  line L238 (6.3479, 39.375) -> (1.0789, 39.375)
  arc A238 (1.0789, 39.375) -> (1.0789, 39.249) centre (1.0789, 39.312) ccw
  line L239 (7.637, 39.249) -> (7.7628, 39.249)
  arc A239 (7.7628, 39.249) -> (7.7628, 39.375) centre (7.7628, 39.312) ccw
  line L240 (7.7628, 39.375) -> (7.637, 39.375)
  arc A240 (7.637, 39.375) -> (7.637, 39.249) centre (7.637, 39.312) ccw
  line L241 (9.0519, 39.249) -> (17.121, 39.249)
  arc A241 (17.121, 39.249) -> (17.121, 39.375) centre (17.121, 39.312) ccw
  line L242 (17.121, 39.375) -> (9.0519, 39.375)
  arc A242 (9.0519, 39.375) -> (9.0519, 39.249) centre (9.0519, 39.312) ccw
  line L243 (1.0789, 39.375) -> (1.9284, 39.375)
  arc A243 (1.9284, 39.375) -> (1.9284, 39.501) centre (1.9284, 39.438) ccw
  line L244 (1.9284, 39.501) -> (1.0789, 39.501)
  arc A244 (1.0789, 39.501) -> (1.0789, 39.375) centre (1.0789, 39.438) ccw
  line L245 (2.8714, 39.375) -> (6.333, 39.375)
  arc A245 (6.333, 39.375) -> (6.333, 39.501) centre (6.333, 39.438) ccw
  line L246 (6.333, 39.501) -> (2.8714, 39.501)
  arc A246 (2.8714, 39.501) -> (2.8714, 39.375) centre (2.8714, 39.438) ccw
  line L247 (7.637, 39.375) -> (7.7628, 39.375)
  arc A247 (7.7628, 39.375) -> (7.7628, 39.501) centre (7.7628, 39.438) ccw
  line L248 (7.7628, 39.501) -> (7.637, 39.501)
  arc A248 (7.637, 39.501) -> (7.637, 39.375) centre (7.637, 39.438) ccw
  line L249 (9.0669, 39.375) -> (17.121, 39.375)
  arc A249 (17.121, 39.375) -> (17.121, 39.501) centre (17.121, 39.438) ccw
  line L250 (17.121, 39.501) -> (9.0669, 39.501)
  arc A250 (9.0669, 39.501) -> (9.0669, 39.375) centre (9.0669, 39.438) ccw
  line L251 (1.0789, 39.501) -> (1.7085, 39.501)
  arc A251 (1.7085, 39.501) -> (1.7085, 39.627) centre (1.7085, 39.564) ccw
  line L252 (1.7085, 39.627) -> (1.0789, 39.627)
  arc A252 (1.0789, 39.627) -> (1.0789, 39.501) centre (1.0789, 39.564) ccw
  line L253 (3.0914, 39.501) -> (7.6365, 39.501)
  arc A253 (7.6365, 39.501) -> (7.6365, 39.627) centre (7.6365, 39.564) ccw
  line L254 (7.6365, 39.627) -> (3.0914, 39.627)
  arc A254 (3.0914, 39.627) -> (3.0914, 39.501) centre (3.0914, 39.564) ccw
  line L255 (7.7634, 39.501) -> (17.121, 39.501)
  arc A255 (17.121, 39.501) -> (17.121, 39.627) centre (17.121, 39.564) ccw
  line L256 (17.121, 39.627) -> (7.7634, 39.627)
  arc A256 (7.7634, 39.627) -> (7.7634, 39.501) centre (7.7634, 39.564) ccw
  line L257 (1.0789, 39.627) -> (1.5825, 39.627)
  arc A257 (1.5825, 39.627) -> (1.5825, 39.753) centre (1.5825, 39.69) ccw
  line L258 (1.5825, 39.753) -> (1.0789, 39.753)
  arc A258 (1.0789, 39.753) -> (1.0789, 39.627) centre (1.0789, 39.69) ccw
  line L259 (3.2174, 39.627) -> (6.333, 39.627)
  arc A259 (6.333, 39.627) -> (6.333, 39.753) centre (6.333, 39.69) ccw
  line L260 (6.333, 39.753) -> (3.2174, 39.753)
  arc A260 (3.2174, 39.753) -> (3.2174, 39.627) centre (3.2174, 39.69) ccw
  line L261 (7.637, 39.627) -> (7.7628, 39.627)
  arc A261 (7.7628, 39.627) -> (7.7628, 39.753) centre (7.7628, 39.69) ccw
  line L262 (7.7628, 39.753) -> (7.637, 39.753)
  arc A262 (7.637, 39.753) -> (7.637, 39.627) centre (7.637, 39.69) ccw
  line L263 (9.0669, 39.627) -> (17.121, 39.627)
  arc A263 (17.121, 39.627) -> (17.121, 39.753) centre (17.121, 39.69) ccw
  line L264 (17.121, 39.753) -> (9.0669, 39.753)
  arc A264 (9.0669, 39.753) -> (9.0669, 39.627) centre (9.0669, 39.69) ccw
  line L265 (1.0789, 39.753) -> (1.4565, 39.753)
  arc A265 (1.4565, 39.753) -> (1.4565, 39.879) centre (1.4565, 39.816) ccw
  line L266 (1.4565, 39.879) -> (1.0789, 39.879)
  arc A266 (1.0789, 39.879) -> (1.0789, 39.753) centre (1.0789, 39.816) ccw
  line L267 (3.3434, 39.753) -> (6.333, 39.753)
  arc A267 (6.333, 39.753) -> (6.333, 39.879) centre (6.333, 39.816) ccw
  line L268 (6.333, 39.879) -> (3.3434, 39.879)
  arc A268 (3.3434, 39.879) -> (3.3434, 39.753) centre (3.3434, 39.816) ccw
  line L269 (7.637, 39.753) -> (7.7628, 39.753)
  arc A269 (7.7628, 39.753) -> (7.7628, 39.879) centre (7.7628, 39.816) ccw
  line L270 (7.7628, 39.879) -> (7.637, 39.879)
  arc A270 (7.637, 39.879) -> (7.637, 39.753) centre (7.637, 39.816) ccw
  line L271 (9.0669, 39.753) -> (17.121, 39.753)
  arc A271 (17.121, 39.753) -> (17.121, 39.879) centre (17.121, 39.816) ccw
  line L272 (17.121, 39.879) -> (9.0669, 39.879)
  arc A272 (9.0669, 39.879) -> (9.0669, 39.753) centre (9.0669, 39.816) ccw
  line L273 (1.0789, 39.879) -> (1.403, 39.879)
  arc A273 (1.403, 39.879) -> (1.403, 40.005) centre (1.403, 39.942) ccw
  line L274 (1.403, 40.005) -> (1.0789, 40.005)
  arc A274 (1.0789, 40.005) -> (1.0789, 39.879) centre (1.0789, 39.942) ccw
  line L275 (3.3968, 39.879) -> (6.3538, 39.879)
  arc A275 (6.3538, 39.879) -> (6.3538, 40.005) centre (6.3538, 39.942) ccw
  line L276 (6.3538, 40.005) -> (3.3968, 40.005)
  arc A276 (3.3968, 40.005) -> (3.3968, 39.879) centre (3.3968, 39.942) ccw
  line L277 (7.637, 39.879) -> (7.7628, 39.879)
  arc A277 (7.7628, 39.879) -> (7.7628, 40.005) centre (7.7628, 39.942) ccw
  line L278 (7.7628, 40.005) -> (7.637, 40.005)
  arc A278 (7.637, 40.005) -> (7.637, 39.879) centre (7.637, 39.942) ccw
  line L279 (9.0462, 39.879) -> (17.121, 39.879)
  arc A279 (17.121, 39.879) -> (17.121, 40.005) centre (17.121, 39.942) ccw
  line L280 (17.121, 40.005) -> (9.0462, 40.005)
  arc A280 (9.0462, 40.005) -> (9.0462, 39.879) centre (9.0462, 39.942) ccw
  line L281 (1.0789, 40.005) -> (1.3509, 40.005)
  arc A281 (1.3509, 40.005) -> (1.3509, 40.131) centre (1.3509, 40.068) ccw
  line L282 (1.3509, 40.131) -> (1.0789, 40.131)
  arc A282 (1.0789, 40.131) -> (1.0789, 40.005) centre (1.0789, 40.068) ccw
  line L283 (3.4489, 40.005) -> (6.406, 40.005)
  arc A283 (6.406, 40.005) -> (6.406, 40.131) centre (6.406, 40.068) ccw
  line L284 (6.406, 40.131) -> (3.4489, 40.131)
  arc A284 (3.4489, 40.131) -> (3.4489, 40.005) centre (3.4489, 40.068) ccw
  line L285 (7.637, 40.005) -> (7.7628, 40.005)
  arc A285 (7.7628, 40.005) -> (7.7628, 40.131) centre (7.7628, 40.068) ccw
  line L286 (7.7628, 40.131) -> (7.637, 40.131)
  arc A286 (7.637, 40.131) -> (7.637, 40.005) centre (7.637, 40.068) ccw
  line L287 (8.994, 40.005) -> (17.121, 40.005)
  arc A287 (17.121, 40.005) -> (17.121, 40.131) centre (17.121, 40.068) ccw
  line L288 (17.121, 40.131) -> (8.994, 40.131)
  arc A288 (8.994, 40.131) -> (8.994, 40.005) centre (8.994, 40.068) ccw
  line L289 (1.0789, 40.131) -> (1.2987, 40.131)
  arc A289 (1.2987, 40.131) -> (1.2987, 40.257) centre (1.2987, 40.194) ccw
  line L290 (1.2987, 40.257) -> (1.0789, 40.257)
  arc A290 (1.0789, 40.257) -> (1.0789, 40.131) centre (1.0789, 40.194) ccw
  line L291 (3.5011, 40.131) -> (6.4582, 40.131)
  arc A291 (6.4582, 40.131) -> (6.4582, 40.257) centre (6.4582, 40.194) ccw
  line L292 (6.4582, 40.257) -> (3.5011, 40.257)
  arc A292 (3.5011, 40.257) -> (3.5011, 40.131) centre (3.5011, 40.194) ccw
  line L293 (7.637, 40.131) -> (7.7628, 40.131)
  arc A293 (7.7628, 40.131) -> (7.7628, 40.257) centre (7.7628, 40.194) ccw
  line L294 (7.7628, 40.257) -> (7.637, 40.257)
  arc A294 (7.637, 40.257) -> (7.637, 40.131) centre (7.637, 40.194) ccw
  line L295 (8.9418, 40.131) -> (17.121, 40.131)
  arc A295 (17.121, 40.131) -> (17.121, 40.257) centre (17.121, 40.194) ccw
  line L296 (17.121, 40.257) -> (8.9418, 40.257)
  arc A296 (8.9418, 40.257) -> (8.9418, 40.131) centre (8.9418, 40.194) ccw
  line L297 (1.0789, 40.257) -> (1.2846, 40.257)
  arc A297 (1.2846, 40.257) -> (1.2846, 40.383) centre (1.2846, 40.32) ccw
  line L298 (1.2846, 40.383) -> (1.0789, 40.383)
  arc A298 (1.0789, 40.383) -> (1.0789, 40.257) centre (1.0789, 40.32) ccw
  line L299 (3.5153, 40.257) -> (6.5104, 40.257)
  arc A299 (6.5104, 40.257) -> (6.5104, 40.383) centre (6.5104, 40.32) ccw
  line L300 (6.5104, 40.383) -> (3.5153, 40.383)
  arc A300 (3.5153, 40.383) -> (3.5153, 40.257) centre (3.5153, 40.32) ccw
  line L301 (7.637, 40.257) -> (7.7628, 40.257)
  arc A301 (7.7628, 40.257) -> (7.7628, 40.383) centre (7.7628, 40.32) ccw
  line L302 (7.7628, 40.383) -> (7.637, 40.383)
  arc A302 (7.637, 40.383) -> (7.637, 40.257) centre (7.637, 40.32) ccw
  line L303 (8.8896, 40.257) -> (17.121, 40.257)
  arc A303 (17.121, 40.257) -> (17.121, 40.383) centre (17.121, 40.32) ccw
  line L304 (17.121, 40.383) -> (8.8896, 40.383)
  arc A304 (8.8896, 40.383) -> (8.8896, 40.257) centre (8.8896, 40.32) ccw
  line L305 (1.0789, 40.383) -> (1.2846, 40.383)
  arc A305 (1.2846, 40.383) -> (1.2846, 40.509) centre (1.2846, 40.446) ccw
  line L306 (1.2846, 40.509) -> (1.0789, 40.509)
  arc A306 (1.0789, 40.509) -> (1.0789, 40.383) centre (1.0789, 40.446) ccw
  line L307 (3.5153, 40.383) -> (6.5928, 40.383)
  arc A307 (6.5928, 40.383) -> (6.5928, 40.509) centre (6.5928, 40.446) ccw
  line L308 (6.5928, 40.509) -> (3.5153, 40.509)
  arc A308 (3.5153, 40.509) -> (3.5153, 40.383) centre (3.5153, 40.446) ccw
  line L309 (7.637, 40.383) -> (7.7628, 40.383)
  arc A309 (7.7628, 40.383) -> (7.7628, 40.509) centre (7.7628, 40.446) ccw
  line L310 (7.7628, 40.509) -> (7.637, 40.509)
  arc A310 (7.637, 40.509) -> (7.637, 40.383) centre (7.637, 40.446) ccw
  line L311 (8.8071, 40.383) -> (17.121, 40.383)
  arc A311 (17.121, 40.383) -> (17.121, 40.509) centre (17.121, 40.446) ccw
  line L312 (17.121, 40.509) -> (8.8071, 40.509)
  arc A312 (8.8071, 40.509) -> (8.8071, 40.383) centre (8.8071, 40.446) ccw
  line L313 (1.0789, 40.509) -> (1.2846, 40.509)
  arc A313 (1.2846, 40.509) -> (1.2846, 40.635) centre (1.2846, 40.572) ccw
  line L314 (1.2846, 40.635) -> (1.0789, 40.635)
  arc A314 (1.0789, 40.635) -> (1.0789, 40.509) centre (1.0789, 40.572) ccw
  line L315 (3.5153, 40.509) -> (6.7188, 40.509)
  arc A315 (6.7188, 40.509) -> (6.7188, 40.635) centre (6.7188, 40.572) ccw
  line L316 (6.7188, 40.635) -> (3.5153, 40.635)
  arc A316 (3.5153, 40.635) -> (3.5153, 40.509) centre (3.5153, 40.572) ccw
  line L317 (7.637, 40.509) -> (7.7628, 40.509)
  arc A317 (7.7628, 40.509) -> (7.7628, 40.635) centre (7.7628, 40.572) ccw
  line L318 (7.7628, 40.635) -> (7.637, 40.635)
  arc A318 (7.637, 40.635) -> (7.637, 40.509) centre (7.637, 40.572) ccw
  line L319 (8.6811, 40.509) -> (17.121, 40.509)
  arc A319 (17.121, 40.509) -> (17.121, 40.635) centre (17.121, 40.572) ccw
  line L320 (17.121, 40.635) -> (8.6811, 40.635)
  arc A320 (8.6811, 40.635) -> (8.6811, 40.509) centre (8.6811, 40.572) ccw
  line L321 (1.0789, 40.635) -> (1.2955, 40.635)
  arc A321 (1.2955, 40.635) -> (1.2955, 40.761) centre (1.2955, 40.698) ccw
  line L322 (1.2955, 40.761) -> (1.0789, 40.761)
  arc A322 (1.0789, 40.761) -> (1.0789, 40.635) centre (1.0789, 40.698) ccw
  line L323 (3.5045, 40.635) -> (6.8448, 40.635)
  arc A323 (6.8448, 40.635) -> (6.8448, 40.761) centre (6.8448, 40.698) ccw
  line L324 (6.8448, 40.761) -> (3.5045, 40.761)
  arc A324 (3.5045, 40.761) -> (3.5045, 40.635) centre (3.5045, 40.698) ccw
  line L325 (7.637, 40.635) -> (7.7628, 40.635)
  arc A325 (7.7628, 40.635) -> (7.7628, 40.761) centre (7.7628, 40.698) ccw
  line L326 (7.7628, 40.761) -> (7.637, 40.761)
  arc A326 (7.637, 40.761) -> (7.637, 40.635) centre (7.637, 40.698) ccw
  line L327 (8.5551, 40.635) -> (17.121, 40.635)
  arc A327 (17.121, 40.635) -> (17.121, 40.761) centre (17.121, 40.698) ccw
  line L328 (17.121, 40.761) -> (8.5551, 40.761)
  arc A328 (8.5551, 40.761) -> (8.5551, 40.635) centre (8.5551, 40.698) ccw
  line L329 (1.0789, 40.761) -> (1.3477, 40.761)
  arc A329 (1.3477, 40.761) -> (1.3477, 40.887) centre (1.3477, 40.824) ccw
  line L330 (1.3477, 40.887) -> (1.0789, 40.887)
  arc A330 (1.0789, 40.887) -> (1.0789, 40.761) centre (1.0789, 40.824) ccw
  line L331 (3.4523, 40.761) -> (7.0348, 40.761)
  arc A331 (7.0348, 40.761) -> (7.0348, 40.887) centre (7.0348, 40.824) ccw
  line L332 (7.0348, 40.887) -> (3.4523, 40.887)
  arc A332 (3.4523, 40.887) -> (3.4523, 40.761) centre (3.4523, 40.824) ccw
  line L333 (7.637, 40.761) -> (7.7628, 40.761)
  arc A333 (7.7628, 40.761) -> (7.7628, 40.887) centre (7.7628, 40.824) ccw
  line L334 (7.7628, 40.887) -> (7.637, 40.887)
  arc A334 (7.637, 40.887) -> (7.637, 40.761) centre (7.637, 40.824) ccw
  line L335 (8.3652, 40.761) -> (17.121, 40.761)
  arc A335 (17.121, 40.761) -> (17.121, 40.887) centre (17.121, 40.824) ccw
  line L336 (17.121, 40.887) -> (8.3652, 40.887)
  arc A336 (8.3652, 40.887) -> (8.3652, 40.761) centre (8.3652, 40.824) ccw
  line L337 (1.0789, 40.887) -> (1.3999, 40.887)
  arc A337 (1.3999, 40.887) -> (1.3999, 41.013) centre (1.3999, 40.95) ccw
  line L338 (1.3999, 41.013) -> (1.0789, 41.013)
  arc A338 (1.0789, 41.013) -> (1.0789, 40.887) centre (1.0789, 40.95) ccw
  line L339 (3.4001, 40.887) -> (7.339, 40.887)
  arc A339 (7.339, 40.887) -> (7.339, 41.013) centre (7.339, 40.95) ccw
  line L340 (7.339, 41.013) -> (3.4001, 41.013)
  arc A340 (3.4001, 41.013) -> (3.4001, 40.887) centre (3.4001, 40.95) ccw
  line L341 (7.637, 40.887) -> (7.7628, 40.887)
  arc A341 (7.7628, 40.887) -> (7.7628, 41.013) centre (7.7628, 40.95) ccw
  line L342 (7.7628, 41.013) -> (7.637, 41.013)
  arc A342 (7.637, 41.013) -> (7.637, 40.887) centre (7.637, 40.95) ccw
  line L343 (8.061, 40.887) -> (17.121, 40.887)
  arc A343 (17.121, 40.887) -> (17.121, 41.013) centre (17.121, 40.95) ccw
  line L344 (17.121, 41.013) -> (8.061, 41.013)
  arc A344 (8.061, 41.013) -> (8.061, 40.887) centre (8.061, 40.95) ccw
  line L345 (1.0789, 41.013) -> (1.452, 41.013)
  arc A345 (1.452, 41.013) -> (1.452, 41.139) centre (1.452, 41.076) ccw
  line L346 (1.452, 41.139) -> (1.0789, 41.139)
  arc A346 (1.0789, 41.139) -> (1.0789, 41.013) centre (1.0789, 41.076) ccw
  line L347 (3.348, 41.013) -> (17.121, 41.013)
  arc A347 (17.121, 41.013) -> (17.121, 41.139) centre (17.121, 41.076) ccw
  line L348 (17.121, 41.139) -> (3.348, 41.139)
  arc A348 (3.348, 41.139) -> (3.348, 41.013) centre (3.348, 41.076) ccw
  line L349 (1.0789, 41.139) -> (1.5746, 41.139)
  arc A349 (1.5746, 41.139) -> (1.5746, 41.265) centre (1.5746, 41.202) ccw
  line L350 (1.5746, 41.265) -> (1.0789, 41.265)
  arc A350 (1.0789, 41.265) -> (1.0789, 41.139) centre (1.0789, 41.202) ccw
  line L351 (3.2253, 41.139) -> (17.121, 41.139)
  arc A351 (17.121, 41.139) -> (17.121, 41.265) centre (17.121, 41.202) ccw
  line L352 (17.121, 41.265) -> (3.2253, 41.265)
  arc A352 (3.2253, 41.265) -> (3.2253, 41.139) centre (3.2253, 41.202) ccw
  line L353 (1.0789, 41.265) -> (1.7006, 41.265)
  arc A353 (1.7006, 41.265) -> (1.7006, 41.391) centre (1.7006, 41.328) ccw
  line L354 (1.7006, 41.391) -> (1.0789, 41.391)
  arc A354 (1.0789, 41.391) -> (1.0789, 41.265) centre (1.0789, 41.328) ccw
  line L355 (3.0993, 41.265) -> (17.121, 41.265)
  arc A355 (17.121, 41.265) -> (17.121, 41.391) centre (17.121, 41.328) ccw
  line L356 (17.121, 41.391) -> (3.0993, 41.391)
  arc A356 (3.0993, 41.391) -> (3.0993, 41.265) centre (3.0993, 41.328) ccw
  line L357 (1.0789, 41.391) -> (1.9094, 41.391)
  arc A357 (1.9094, 41.391) -> (1.9094, 41.517) centre (1.9094, 41.454) ccw
  line L358 (1.9094, 41.517) -> (1.0789, 41.517)
  arc A358 (1.0789, 41.517) -> (1.0789, 41.391) centre (1.0789, 41.454) ccw
  line L359 (2.8906, 41.391) -> (17.121, 41.391)
  arc A359 (17.121, 41.391) -> (17.121, 41.517) centre (17.121, 41.454) ccw
  line L360 (17.121, 41.517) -> (2.8906, 41.517)
  arc A360 (2.8906, 41.517) -> (2.8906, 41.391) centre (2.8906, 41.454) ccw
  line L361 (1.0789, 41.517) -> (17.121, 41.517)
  arc A361 (17.121, 41.517) -> (17.121, 41.643) centre (17.121, 41.58) ccw
  line L362 (17.121, 41.643) -> (1.0789, 41.643)
  arc A362 (1.0789, 41.643) -> (1.0789, 41.517) centre (1.0789, 41.58) ccw
  line L363 (1.0789, 41.643) -> (17.121, 41.643)
  arc A363 (17.121, 41.643) -> (17.121, 41.769) centre (17.121, 41.706) ccw
  line L364 (17.121, 41.769) -> (1.0789, 41.769)
  arc A364 (1.0789, 41.769) -> (1.0789, 41.643) centre (1.0789, 41.706) ccw
  line L365 (1.0789, 41.769) -> (17.121, 41.769)
  arc A365 (17.121, 41.769) -> (17.121, 41.895) centre (17.121, 41.832) ccw
  line L366 (17.121, 41.895) -> (1.0789, 41.895)
  arc A366 (1.0789, 41.895) -> (1.0789, 41.769) centre (1.0789, 41.832) ccw
  line L367 (1.0789, 41.895) -> (17.121, 41.895)
  arc A367 (17.121, 41.895) -> (17.121, 42.021) centre (17.121, 41.958) ccw
  line L368 (17.121, 42.021) -> (1.0789, 42.021)
  arc A368 (1.0789, 42.021) -> (1.0789, 41.895) centre (1.0789, 41.958) ccw
  line L369 (1.0789, 42.021) -> (17.121, 42.021)
  arc A369 (17.121, 42.021) -> (17.121, 42.147) centre (17.121, 42.084) ccw
  line L370 (17.121, 42.147) -> (1.0789, 42.147)
  arc A370 (1.0789, 42.147) -> (1.0789, 42.021) centre (1.0789, 42.084) ccw
  line L371 (1.0789, 42.147) -> (17.121, 42.147)
  arc A371 (17.121, 42.147) -> (17.121, 42.273) centre (17.121, 42.21) ccw
  line L372 (17.121, 42.273) -> (1.0789, 42.273)
  arc A372 (1.0789, 42.273) -> (1.0789, 42.147) centre (1.0789, 42.21) ccw
  line L373 (1.0789, 42.273) -> (17.121, 42.273)
  arc A373 (17.121, 42.273) -> (17.121, 42.399) centre (17.121, 42.336) ccw
  line L374 (17.121, 42.399) -> (1.0789, 42.399)
  arc A374 (1.0789, 42.399) -> (1.0789, 42.273) centre (1.0789, 42.336) ccw
  line L375 (1.0789, 42.399) -> (17.121, 42.399)
  arc A375 (17.121, 42.399) -> (17.121, 42.525) centre (17.121, 42.462) ccw
  line L376 (17.121, 42.525) -> (1.0789, 42.525)
  arc A376 (1.0789, 42.525) -> (1.0789, 42.399) centre (1.0789, 42.462) ccw
  line L377 (1.0789, 42.525) -> (17.121, 42.525)
  arc A377 (17.121, 42.525) -> (17.121, 42.651) centre (17.121, 42.588) ccw
  line L378 (17.121, 42.651) -> (1.0789, 42.651)
  arc A378 (1.0789, 42.651) -> (1.0789, 42.525) centre (1.0789, 42.588) ccw
  line L379 (1.0789, 42.651) -> (17.121, 42.651)
  arc A379 (17.121, 42.651) -> (17.121, 42.777) centre (17.121, 42.714) ccw
  line L380 (17.121, 42.777) -> (1.0789, 42.777)
  arc A380 (1.0789, 42.777) -> (1.0789, 42.651) centre (1.0789, 42.714) ccw
  line L381 (1.0789, 42.777) -> (1.8995, 42.777)
  arc A381 (1.8995, 42.777) -> (1.8995, 42.903) centre (1.8995, 42.84) ccw
  line L382 (1.8995, 42.903) -> (1.0789, 42.903)
  arc A382 (1.0789, 42.903) -> (1.0789, 42.777) centre (1.0789, 42.84) ccw
  line L383 (2.337, 42.777) -> (2.4628, 42.777)
  arc A383 (2.4628, 42.777) -> (2.4628, 42.903) centre (2.4628, 42.84) ccw
  line L384 (2.4628, 42.903) -> (2.337, 42.903)
  arc A384 (2.337, 42.903) -> (2.337, 42.777) centre (2.337, 42.84) ccw
  line L385 (2.9003, 42.777) -> (17.121, 42.777)
  arc A385 (17.121, 42.777) -> (17.121, 42.903) centre (17.121, 42.84) ccw
  line L386 (17.121, 42.903) -> (2.9003, 42.903)
  arc A386 (2.9003, 42.903) -> (2.9003, 42.777) centre (2.9003, 42.84) ccw
  line L387 (1.0789, 42.903) -> (1.6629, 42.903)
  arc A387 (1.6629, 42.903) -> (1.6629, 43.029) centre (1.6629, 42.966) ccw
  line L388 (1.6629, 43.029) -> (1.0789, 43.029)
  arc A388 (1.0789, 43.029) -> (1.0789, 42.903) centre (1.0789, 42.966) ccw
  line L389 (2.337, 42.903) -> (2.4628, 42.903)
  arc A389 (2.4628, 42.903) -> (2.4628, 43.029) centre (2.4628, 42.966) ccw
  line L390 (2.4628, 43.029) -> (2.337, 43.029)
  arc A390 (2.337, 43.029) -> (2.337, 42.903) centre (2.337, 42.966) ccw
  line L391 (3.137, 42.903) -> (17.121, 42.903)
  arc A391 (17.121, 42.903) -> (17.121, 43.029) centre (17.121, 42.966) ccw
  line L392 (17.121, 43.029) -> (3.137, 43.029)
  arc A392 (3.137, 43.029) -> (3.137, 42.903) centre (3.137, 42.966) ccw
  line L393 (1.0789, 43.029) -> (1.5369, 43.029)
  arc A393 (1.5369, 43.029) -> (1.5369, 43.155) centre (1.5369, 43.092) ccw
  line L394 (1.5369, 43.155) -> (1.0789, 43.155)
  arc A394 (1.0789, 43.155) -> (1.0789, 43.029) centre (1.0789, 43.092) ccw